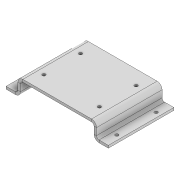
# Autodesk Inventor part: BaseMotor
Saved by Autodesk Inventor 2021 (Build 250183000, 183)
## iProperties
Created: 2021-08-18
Part Number: BaseMotor
Material: Generic
Document SubType Name: Sheet Metal
Designer: Santiago Suárez
Density: 1 g/cm^3
Sheet Metal Rule: Default_mm
Appearance: Default
Flat Pattern Width: 47.1954 cm
Flat Pattern Length: 25 cm
Flat Pattern Area: 1179.88 cm^2
Sheet Metal Width: 471.954 mm
Sheet Metal Length: 250.000 mm
Sheet Metal Area: 117988.494 mm^2
Author: Santiago Suárez
Autodesk Inventor part; units mm, degrees
ref_plane "YZ Plane" through (0, 0, 0) normal (1, 0, 0) x (0, 1, 0)
ref_plane "XZ Plane" through (0, 0, 0) normal (0, 1, 0) x (-1, 0, 0)
ref_plane "XY Plane" through (0, 0, 0) normal (0, 0, 1) x (1, 0, 0)
sketch "Sketch1" plane through (0, 0, 0) normal (0, 1, 0) x (-1, 0, 0)
  line L0 (150, 125) -> (-150, 125)
  line L1 (-150, 125) -> (-150, -125)
  line L2 (-150, -125) -> (150, -125)
  line L3 (150, -125) -> (150, 125)
  point P0 (0, 0)
  dimension "d0" = 300
  dimension "d1" = 250
  dimension "d2" = 125
  dimension "d29" = 150
  measures "d0" distance of L0.start L0.end
  measures "d1" distance of L2.end L0.start
  measures "d2" distance from line of L0 point (0, 0)
  measures "d29" distance from line of L3 point (0, 0)
extrude "Plate1" add sketch "Sketch1" along normal blind 9.5
sketch "Sketch4" plane through (0, 9.5, 0) normal (0, 1, 0) x (1, 0, 0)
  line L0 (-106, -70) -> (106, -70)
  line L1 (106, -70) -> (106, 70)
  line L2 (106, 70) -> (-106, 70)
  line L3 (-106, 70) -> (-106, -70)
  line L4 (-150, -125) -> (-150, 125) projected
  point P0 (0, 0)
  point P1 (-130, -106)
  point P2 (-130, 106)
  dimension "d24" = 140
  dimension "d25" = 212
  dimension "d27" = 70
  dimension "d28" = 106
  constraints: 8 end point, 4 coincident, 2 parallel, 1 horizontal, 1 perpendicular, 1 other
  measures "d24" distance of L2.end L0.start
  measures "d25" distance of L0.start L0.end
  measures "d27" distance from line of point (0, 0) L0
  measures "d28" distance from line of point (0, 0) L3
hole "Hole1" at (-106, 9.5, 70) at (-106, 9.5, -70) at (106, 9.5, 70) at (106, 9.5, -70) direction (0, -1, 0) diameter 12 depth 9.5
sketch "Sketch8" plane through (-140.5, 9.5, 125) normal (-1, 0, 0) x (0, 1, 0)
  line L0 (0, -250) -> (0, 0)
  line L1 (0, 0) -> (-64.5, 0)
  line L2 (-64.5, 0) -> (-64.5, -250)
  line L3 (-64.5, -250) -> (0, -250)
  constraints: 6 end point, 1 horizontal, 1 perpendicular, 1 vertical
edge flange "Flange5" height 64.5 angle 90 thickness 9.5 bend radius 9.5 thickness toward (-1, 0, 0) relief straight relief width 9.5 relief depth 4.75 edges at (-150, 9.5, 0) wall of the first edge with corners at (-140.5, 9.5, -125) (-140.5, 9.5, 125) (-140.5, -55, 125) (-140.5, -55, -125)
bend "Bend5"
corner "Corner5"
sketch "Sketch9" plane through (140.5, 9.5, -125) normal (1, 0, 0) x (0, -1, 0)
  line L0 (0, 250) -> (0, 0)
  line L1 (0, 0) -> (64.5, 0)
  line L2 (64.5, 0) -> (64.5, 250)
  line L3 (64.5, 250) -> (0, 250)
  constraints: 6 end point, 1 horizontal, 1 perpendicular, 1 vertical
edge flange "Flange6" height 64.5 angle 90 thickness 9.5 bend radius 9.5 thickness toward (1, 0, 0) relief straight relief width 9.5 relief depth 4.75 edges at (150, 9.5, 0) wall of the first edge with corners at (140.5, 9.5, 125) (140.5, 9.5, -125) (140.5, -55, -125) (140.5, -55, 125)
bend "Bend6"
corner "Corner6"
sketch "Sketch10" plane through (-140.5, -45.5, -125) normal (0, -1, 0) x (-1, 0, 0)
  line L0 (0, 250) -> (0, 0)
  line L1 (0, 0) -> (54.5, 0)
  line L2 (54.5, 0) -> (54.5, 250)
  line L3 (54.5, 250) -> (0, 250)
  constraints: 6 end point, 1 horizontal, 1 perpendicular, 1 vertical
edge flange "Flange7" height 45 angle 90 thickness 9.5 bend radius 9.5 thickness toward (0, -1, 0) relief straight relief width 9.5 relief depth 4.75 edges at (-140.5, -55, 0) wall of the first edge with corners at (-140.5, -45.5, 125) (-140.5, -45.5, -125) (-195, -45.5, -125) (-195, -45.5, 125)
bend "Bend7"
corner "Corner7"
sketch "Sketch11" plane through (140.5, -45.5, 125) normal (0, -1, 0) x (-1, 0, 0)
  line L0 (0, -250) -> (0, 0)
  line L1 (0, 0) -> (-54.5, 0)
  line L2 (-54.5, 0) -> (-54.5, -250)
  line L3 (-54.5, -250) -> (0, -250)
  constraints: 6 end point, 1 horizontal, 1 perpendicular, 1 vertical
edge flange "Flange8" height 45 angle 90 thickness 9.5 bend radius 9.5 thickness toward (0, -1, 0) relief straight relief width 9.5 relief depth 4.75 edges at (140.5, -55, 0) wall of the first edge with corners at (140.5, -45.5, -125) (140.5, -45.5, 125) (195, -45.5, 125) (195, -45.5, -125)
bend "Bend8"
corner "Corner8"
sketch "Sketch12" plane through (-195, -45.5, 125) normal (0, 1, 0) x (1, 0, 0)
  line L0 (35.5, 250) -> (0, 250) projected
  line L1 (17.75, 250) -> (17.75, 0)
  line L2 (35.5, 0) -> (0, 0) projected
  line L3 (0, 0) -> (0, 250) projected
  line L4 (0, 200) -> (35.5, 200)
  line L5 (0, 50) -> (35.5, 50)
  line L6 (35.5, 250) -> (35.5, 0) projected
  point P0 (195, 125)
  point P1 (17.75, 200)
  point P2 (17.75, 50)
  dimension "d110" = 50
  dimension "d111" = 50
  constraints: 6 end point, 4 midpoint, 3 point on line, 2 horizontal
  measures "d110" distance between parallel lines of L2 L5
  measures "d111" distance between parallel lines of L0 L4
hole "Hole3" at (-177.25, -45.5, -75) at (-177.25, -45.5, 75) direction (0, -1, 0) diameter 12 depth 9.5
mirror "Mirror2" about plane through (0, 0, 0) normal (1, 0, 0) of "Hole3"
equation "\"d28\" = 0.5 * d25"
equation "\"d35\" = Thickness"
equation "\"d117\" = Thickness"
equation "\"d3\" = Thickness"
equation "\"d69\" = BendReliefWidth"
equation "\"d70\" = BendReliefDepth"
equation "\"d71\" = MinimumRemnant"
equation "\"d72\" = TransitionRadius"
equation "\"d75\" = BendRadius"
equation "\"d76\" = CornerReliefSize"
equation "\"d77\" = GapSize"
equation "\"d78\" = JacobiRadiusSize"
equation "\"d79\" = BendReliefWidth"
equation "\"d80\" = BendReliefDepth"
equation "\"d81\" = MinimumRemnant"
equation "\"d82\" = TransitionRadius"
equation "\"d85\" = BendRadius"
equation "\"d86\" = CornerReliefSize"
equation "\"d87\" = GapSize"
equation "\"d88\" = JacobiRadiusSize"
equation "\"d89\" = BendReliefWidth"
equation "\"d90\" = BendReliefDepth"
equation "\"d91\" = MinimumRemnant"
equation "\"d92\" = TransitionRadius"
equation "\"d95\" = BendRadius"
equation "\"d96\" = CornerReliefSize"
equation "\"d97\" = GapSize"
equation "\"d98\" = JacobiRadiusSize"
equation "\"d99\" = BendReliefWidth"
equation "\"d100\" = BendReliefDepth"
equation "\"d101\" = MinimumRemnant"
equation "\"d102\" = TransitionRadius"
equation "\"d105\" = BendRadius"
equation "\"d106\" = CornerReliefSize"
equation "\"d107\" = GapSize"
equation "\"d108\" = JacobiRadiusSize"
equation "\"d2\" = 0.5 * d1"
equation "\"d29\" = 0.5 * d0"
equation "\"BendRadius\" = Thickness"
equation "\"BendReliefWidth\" = Thickness"
equation "\"BendReliefDepth\" = 0.5 * Thickness"
equation "\"CornerReliefSize\" = 4 * Thickness"
equation "\"MinimumRemnant\" = 2 * Thickness"
equation "\"TransitionRadius\" = BendRadius"
equation "\"JacobiRadiusSize\" = BendRadius"
equation "\"GapSize\" = Thickness"
equation "\"Thickness\" = 9.5"
body "Solid1"
